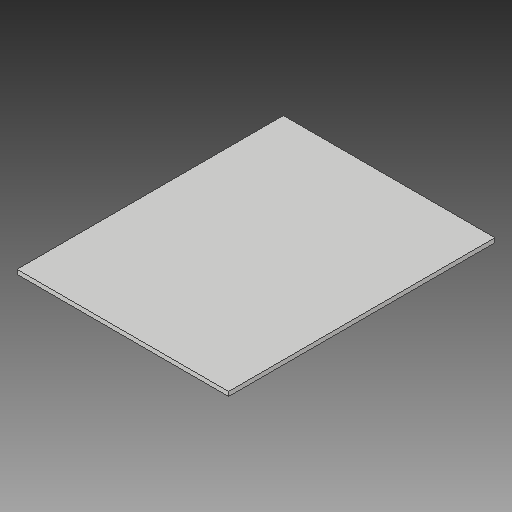
# Autodesk Inventor part: Plywood base - sax.0005
Saved by Autodesk Inventor 2018.2 (Build 222227000, 227)
## iProperties
Created: 2018-01-30
Material: Generic
Document SubType Name: Modeling
Designer: owner
Density: 1 g/cm^3
Appearance: Default
Author: owner
Autodesk Inventor part; units mm, degrees
ref_plane "YZ Plane" through (0, 0, 0) normal (1, 0, 0) x (0, 1, 0)
ref_plane "XZ Plane" through (0, 0, 0) normal (0, 1, 0) x (-1, 0, 0)
ref_plane "XY Plane" through (0, 0, 0) normal (0, 0, 1) x (1, 0, 0)
sketch "Sketch1" plane through (0, 0, 0) normal (0, 0, 1) x (1, 0, 0)
  line L0 (0, 0) -> (927.4048, 0)
  line L1 (927.4048, 0) -> (927.4048, 19.05)
  line L2 (927.4048, 19.05) -> (0, 19.05)
  line L3 (0, 19.05) -> (0, 0)
  line L4 (0.0889, 17.7165) -> (0, 17.7165)
  ellipse E0 centre (11.1959, 23.2341) end of major axis (1.455, 23.2335) minor radius 0.0002 (16.0493, 23.2346) -> (6.3425, 23.2336) ccw projected
  ellipse E1 centre (11.1961, 19.0177) end of major axis (1.4552, 19.0171) minor radius 0.0002 (16.0495, 19.0182) -> (6.3428, 19.0172) ccw projected
  dimension "d0" = 927.4048
  dimension "d1" = 19.05
  constraints: 10 end point, 3 perpendicular, 1 horizontal, 1 parallel, 1 point on line, 2 other
  measures "d0" distance of L0.start L0.end
  measures "d1" distance of L0.end L1.end
extrude "Extrusion1" add sketch "Sketch1" against normal blind 1167.4602
body "Solid1"
